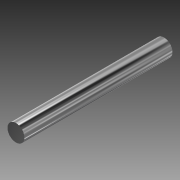
# Autodesk Inventor part: pinSDCARDTOTEENSY
Saved by Autodesk Inventor 2014 (Build 180170000, 170)
## iProperties
Created: 2014-06-01
Part Number: pinSDCARDTOTEENSY
Material: Nickel-Copper Alloy 400
Document SubType Name: Modeling
Designer: jose
Mass: 0.0310691 g
Surface Area: 0.185982 cm^2
Volume: 0.00351858 cm^3
Density: 8.83 g/cm^3
Appearance: Chrome - Polished
Author: jose
Autodesk Inventor part; units mm, degrees
ref_plane "YZ Plane" through (0, 0, 0) normal (1, 0, 0) x (0, 1, 0)
ref_plane "XZ Plane" through (0, 0, 0) normal (0, 1, 0) x (-1, 0, 0)
ref_plane "XY Plane" through (0, 0, 0) normal (0, 0, 1) x (1, 0, 0)
sketch "Sketch1" plane through (0, 0, 0) normal (0, 1, 0) x (-1, 0, 0)
  circle A0 centre (0, 0) radius 0.4
  dimension "d0" = 0.8
  constraints: 1 centre point, 1 coincident
  measures "d0" diameter of A0
extrude "Extrusion1" add sketch "Sketch1" along normal mid plane 7
body "Solid1"
